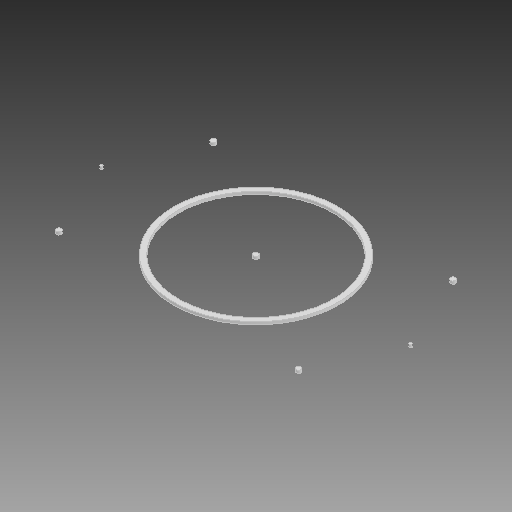
# Autodesk Inventor part: Metkes_1
Saved by Autodesk Inventor 2023 (Build 270158000, 158)
## iProperties
Created: 2022-01-17
Part Number: Metkes_1
Material: Типовые
Document SubType Name: Modeling
Designer: Администратор
Density: 1 g/cm^3
Appearance: По умолчанию
Author: Администратор
Autodesk Inventor part; units mm, degrees
ref_plane "YZ Plane" through (0, 0, 0) normal (1, 0, 0) x (0, 1, 0)
ref_plane "XZ Plane" through (0, 0, 0) normal (0, 1, 0) x (-1, 0, 0)
ref_plane "XY Plane" through (0, 0, 0) normal (0, 0, 1) x (1, 0, 0)
sketch "Эскиз1" plane through (0, 0, 0) normal (0, 1, 0) x (-1, 0, 0)
  circle A0 centre (0, 0) radius 300
  circle A1 centre (0, 0) radius 320
  circle A2 centre (465, -300) radius 10
  line L0 (915, -610) -> (-915, -610)
  line L1 (-915, -610) -> (-915, 610)
  line L2 (-915, 610) -> (915, 610)
  line L3 (915, 610) -> (915, -610)
  line L4 (0, -610) -> (0, 610) construction
  line L5 (915, 0) -> (-915, 0) construction
  circle A3 centre (465, 300) radius 10
  circle A4 centre (-465, -300) radius 10
  circle A5 centre (-465, 300) radius 10
  circle A6 centre (0, 0) radius 10
  circle A7 centre (600, 0) radius 5
  circle A8 centre (-600, 0) radius 5
  dimension "d0" = 600
  dimension "d1" = 20
  dimension "d2" = 20
  dimension "d3" = 450
  dimension "d4" = 310
  dimension "d5" = 1830
  dimension "d6" = 1220
  dimension "d12" = 10
  dimension "d13" = 600
  constraints: 12 end point, 9 centre point, 5 midpoint, 4 symmetric about line, 3 coincident, 2 parallel, 1 equal radius, 1 horizontal, 1 perpendicular, 1 point on line, 4 other
  measures "d0" diameter of A0
  measures "d1" radial gap between concentric circles of A0 A1
  measures "d2" diameter of A2
  measures "d3" distance from line of L3 A2.centre
  measures "d4" distance from line of L0 A2.centre
  measures "d5" distance of L0.start L0.end
  measures "d6" distance of L2.end L0.start
  measures "d12" diameter of A7
  measures "d13" distance of point (0, 0) A7.centre
extrude "Выдавливание1" add sketch "Эскиз1" along normal blind 10.5 contours A1 | A2 | A3 | A4 | A5 | A6 | A7 | A8
